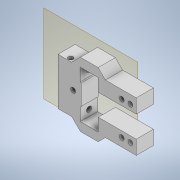
# Autodesk Inventor part: 30_Cube_Cube_Z_Focus_MGN_NEMA_belt_pushing_slide_v3
Saved by Autodesk Inventor 2022 (Build 260153000, 153)
## iProperties
Created: 2021-12-20
Part Number: 30_Cube_Cube_Z_Focus_MGN_NEMA_belt_pushing_slide_v3
Material: Generisch
Document SubType Name: Modeling
Designer: diederichbenedict
Density: 1 g/cm^3
Appearance: Vorgabe
Author: diederichbenedict
Autodesk Inventor part; units mm, degrees
ref_plane "YZ Plane" through (0, 0, 0) normal (1, 0, 0) x (0, 1, 0)
ref_plane "XZ Plane" through (0, 0, 0) normal (0, 1, 0) x (-1, 0, 0)
ref_plane "XY Plane" through (0, 0, 0) normal (0, 0, 1) x (1, 0, 0)
ref_plane "Arbeitsebene1" through (0, 0, 0) normal (0, 0, 1) x (1, 0, 0)
sketch "Skizze1" plane through (0, 0, 0) normal (0, 0, 1) x (1, 0, 0)
  arc A0 (12.7966, 13.5152) -> (12.2972, 14.0928) centre (11.6862, 13.06) ccw construction
  arc A1 (12.1755, 14.2862) -> (12.2972, 14.0928) centre (12.4245, 14.308) ccw construction
  line L0 (12.1755, 14.2862) -> (12.1453, 14.6318) construction
  arc A2 (12.1453, 14.6318) -> (11.8962, 14.86) centre (11.8962, 14.61) ccw construction
  line L1 (11.8962, 14.86) -> (11.4438, 14.86) construction
  arc A3 (11.4438, 14.86) -> (11.1947, 14.6318) centre (11.4438, 14.61) ccw construction
  line L2 (11.1947, 14.6318) -> (11.1627, 14.2652) construction
  arc A4 (11.0468, 14.0755) -> (11.1627, 14.2652) centre (10.9136, 14.287) ccw construction
  arc A5 (11.0468, 14.0755) -> (10.5759, 13.5152) centre (11.6862, 13.06) ccw construction
  arc A6 (10.3446, 13.36) -> (10.5759, 13.5152) centre (10.3446, 13.61) ccw construction
  line L3 (10.3446, 13.36) -> (9.67, 13.36) construction
  line L4 (9.67, 13.36) -> (9.17, 13.86) construction
  line L5 (9.17, 13.86) -> (9.17, 24.86) construction
  line L6 (9.17, 24.86) -> (9.67, 25.36) construction
  line L7 (9.67, 25.36) -> (10.3446, 25.36) construction
  arc A7 (10.5759, 25.2048) -> (10.3446, 25.36) centre (10.3446, 25.11) ccw construction
  arc A8 (10.5759, 25.2048) -> (11.0468, 24.6445) centre (11.6862, 25.66) ccw construction
  arc A9 (11.1627, 24.4548) -> (11.0468, 24.6445) centre (10.9136, 24.433) ccw construction
  line L8 (11.1627, 24.4548) -> (11.1947, 24.0882) construction
  arc A10 (11.1947, 24.0882) -> (11.4438, 23.86) centre (11.4438, 24.11) ccw construction
  line L9 (11.4438, 23.86) -> (11.8962, 23.86) construction
  arc A11 (11.8962, 23.86) -> (12.1453, 24.0882) centre (11.8962, 24.11) ccw construction
  line L10 (12.1453, 24.0882) -> (12.1755, 24.4338) construction
  arc A12 (12.2972, 24.6272) -> (12.1755, 24.4338) centre (12.4245, 24.412) ccw construction
  arc A13 (12.2972, 24.6272) -> (12.7966, 25.2048) centre (11.6862, 25.66) ccw construction
  arc A14 (13.0279, 25.36) -> (12.7966, 25.2048) centre (13.0279, 25.11) ccw construction
  line L11 (13.0279, 25.36) -> (14.17, 25.36) construction
  line L12 (14.17, 25.36) -> (14.17, 32.26) construction
  line L13 (14.17, 32.26) -> (13.57, 32.86) construction
  line L14 (13.57, 32.86) -> (10.17, 32.86) construction
  arc A15 (9.37, 32.86) -> (10.17, 32.86) centre (9.77, 33.16) ccw construction
  line L15 (9.37, 32.86) -> (4.77, 32.86) construction
  line L16 (4.77, 32.86) -> (4.17, 32.26) construction
  line L17 (4.17, 32.26) -> (4.17, 25.76) construction
  line L18 (4.17, 25.76) -> (4.57, 25.36) construction
  line L19 (4.57, 25.36) -> (4.57, 13.36) construction
  line L20 (4.57, 13.36) -> (4.17, 12.96) construction
  line L21 (4.17, 12.96) -> (4.17, 6.46) construction
  line L22 (4.17, 6.46) -> (4.77, 5.86) construction
  line L23 (4.77, 5.86) -> (13.57, 5.86) construction
  line L24 (13.57, 5.86) -> (14.17, 6.46) construction
  line L25 (14.17, 6.46) -> (14.17, 13.36) construction
  line L26 (14.17, 13.36) -> (13.0279, 13.36) construction
  arc A16 (12.7966, 13.5152) -> (13.0279, 13.36) centre (13.0279, 13.61) ccw construction
  line L27 (13.6528, 5.66) -> (4.6872, 5.66) construction
  line L28 (4.6872, 5.66) -> (3.97, 6.3772) construction
  line L29 (3.97, 6.3772) -> (3.97, 13.0428) construction
  line L30 (3.97, 13.0428) -> (4.37, 13.4428) construction
  line L31 (4.37, 13.4428) -> (4.37, 25.2772) construction
  line L32 (4.37, 25.2772) -> (3.97, 25.6772) construction
  line L33 (3.97, 25.6772) -> (3.97, 32.3428) construction
  line L34 (3.97, 32.3428) -> (4.6872, 33.06) construction
  line L35 (4.6872, 33.06) -> (9.4872, 33.06) construction
  arc A17 (9.4872, 33.06) -> (10.0528, 33.06) centre (9.77, 33.16) ccw construction
  line L36 (10.0528, 33.06) -> (13.6528, 33.06) construction
  line L37 (13.6528, 33.06) -> (14.37, 32.3428) construction
  line L38 (14.37, 32.3428) -> (14.37, 25.16) construction
  line L39 (14.37, 25.16) -> (13.0279, 25.16) construction
  arc A18 (13.0279, 25.16) -> (12.9816, 25.129) centre (13.0279, 25.11) ccw construction
  arc A19 (12.3991, 24.4551) -> (12.9816, 25.129) centre (11.6862, 25.66) ccw construction
  arc A20 (12.3991, 24.4551) -> (12.3747, 24.4164) centre (12.4245, 24.412) ccw construction
  line L40 (12.3747, 24.4164) -> (12.3445, 24.0708) construction
  arc A21 (11.8962, 23.66) -> (12.3445, 24.0708) centre (11.8962, 24.11) ccw construction
  line L41 (11.8962, 23.66) -> (11.4438, 23.66) construction
  arc A22 (10.9955, 24.0708) -> (11.4438, 23.66) centre (11.4438, 24.11) ccw construction
  line L42 (10.9955, 24.0708) -> (10.9634, 24.4373) construction
  arc A23 (10.9634, 24.4373) -> (10.9403, 24.4753) centre (10.9136, 24.433) ccw construction
  arc A24 (10.3909, 25.129) -> (10.9403, 24.4753) centre (11.6862, 25.66) ccw construction
  arc A25 (10.3909, 25.129) -> (10.3446, 25.16) centre (10.3446, 25.11) ccw construction
  line L43 (10.3446, 25.16) -> (9.7528, 25.16) construction
  line L44 (9.7528, 25.16) -> (9.37, 24.7772) construction
  line L45 (9.37, 24.7772) -> (9.37, 13.9428) construction
  line L46 (9.37, 13.9428) -> (9.7528, 13.56) construction
  line L47 (9.7528, 13.56) -> (10.3446, 13.56) construction
  arc A26 (10.3446, 13.56) -> (10.3909, 13.591) centre (10.3446, 13.61) ccw construction
  arc A27 (10.9403, 14.2447) -> (10.3909, 13.591) centre (11.6862, 13.06) ccw construction
  arc A28 (10.9403, 14.2447) -> (10.9634, 14.2827) centre (10.9136, 14.287) ccw construction
  line L48 (10.9634, 14.2827) -> (10.9955, 14.6492) construction
  arc A29 (11.4438, 15.06) -> (10.9955, 14.6492) centre (11.4438, 14.61) ccw construction
  line L49 (11.4438, 15.06) -> (11.8962, 15.06) construction
  arc A30 (12.3445, 14.6492) -> (11.8962, 15.06) centre (11.8962, 14.61) ccw construction
  line L50 (12.3445, 14.6492) -> (12.3747, 14.3036) construction
  arc A31 (12.3747, 14.3036) -> (12.3991, 14.2649) centre (12.4245, 14.308) ccw construction
  arc A32 (12.9816, 13.591) -> (12.3991, 14.2649) centre (11.6862, 13.06) ccw construction
  arc A33 (12.9816, 13.591) -> (13.0279, 13.56) centre (13.0279, 13.61) ccw construction
  line L51 (13.0279, 13.56) -> (14.37, 13.56) construction
  line L52 (14.37, 13.56) -> (14.37, 6.3772) construction
  line L53 (14.37, 6.3772) -> (13.6528, 5.66) construction
  line L54 (16.97, 24.8315) -> (24.85, 24.8315) construction
  line L55 (24.85, 36.23) -> (20.77, 36.23) construction
  line L56 (20.77, 36.23) -> (16.87, 36.23) construction
  line L57 (14.37, 25.66) -> (36.4731, 25.66)
  line L58 (14.37, 25.66) -> (36.4731, 25.66) construction
  line L59 (36.4731, 25.66) -> (36.4731, 33.86)
  line L60 (36.4731, 33.86) -> (18.5197, 33.86)
  line L61 (18.5197, 33.86) -> (14.3197, 38.06)
  line L62 (14.3197, 38.06) -> (3.97, 38.06)
  line L63 (-9.03, 33.06) -> (-9.03, 19.36)
  line L64 (-9.03, 19.36) -> (4.37, 19.36)
  line L65 (4.37, 19.36) -> (4.37, 25.2772)
  line L66 (4.37, 25.2772) -> (3.97, 25.6772)
  line L67 (3.97, 25.6772) -> (3.97, 33.06)
  line L68 (3.97, 33.06) -> (14.37, 33.06)
  line L69 (14.37, 33.06) -> (14.37, 25.66)
  circle A34 centre (-3.43, 19.36) radius 1.75 construction
  circle A35 centre (-0.2031, 19.36) radius 1.4
  circle A36 centre (60.62, 30.4425) radius 2.45 projected
  circle A37 centre (35.7803, 19.36) radius 2.45 projected
  circle A38 centre (60.62, 8.3286) radius 2.45 projected
  line L70 (29.0574, 13.415) -> (26.7455, 13.415) projected
  line L71 (26.7455, 13.415) -> (26.7455, 10.1303) projected
  arc A39 (26.7455, 9.327) -> (26.7455, 10.1303) centre (28.0867, 9.7286) ccw projected
  line L72 (26.7455, 9.327) -> (26.7455, 5.8628) projected
  line L73 (26.7455, 5.8628) -> (35.12, 4.36) projected
  line L74 (35.12, 4.36) -> (65.12, 4.36) projected
  line L75 (65.12, 4.36) -> (65.12, 34.36) projected
  line L76 (65.12, 34.36) -> (35.12, 34.36) projected
  line L77 (35.12, 34.36) -> (26.7455, 32.9029) projected
  line L78 (26.7455, 32.9029) -> (26.7455, 29.4442) projected
  arc A40 (26.7455, 28.6409) -> (26.7455, 29.4442) centre (28.0867, 29.0425) ccw projected
  line L79 (26.7455, 28.6409) -> (26.7455, 25.3561) projected
  line L80 (26.7455, 25.3561) -> (29.0574, 25.3561) projected
  line L81 (29.0574, 25.3561) -> (29.0574, 13.415) projected
  circle A41 centre (50.12, 19.36) radius 10.5 projected
  circle A42 centre (33.0867, 29.0425) radius 1.4 projected
  circle A43 centre (33.0867, 9.7286) radius 1.4 projected
  line L82 (36.7731, 34.36) -> (36.7731, 25.3561) projected
  line L83 (36.7731, 13.415) -> (36.7731, 4.36) projected
  circle A44 centre (33.0867, 29.0425) radius 1.4
  circle A45 centre (28.0867, 29.0425) radius 1.4
  line L84 (3.97, 38.06) -> (-1.03, 33.06)
  line L85 (3.97, 38.06) -> (11.0411, 38.06) construction
  line L86 (-1.03, 33.06) -> (-9.03, 33.06)
  point P0 (0, 0)
  point P1 (1.1969, 19.36)
  point P2 (-1.6031, 19.36)
  dimension "d0" = 0.2
  dimension "d2" = 5
  dimension "d4" = 13
  dimension "d5" = 2.8
  dimension "d7" = 0.5
  dimension "d8" = 3.5
  dimension "d19" = 0.3
  dimension "d20" = 0.5
  dimension "d21" = 135
  dimension "d28" = 8.8269
  constraints: 86 end point, 36 point on circle, 20 centre point, 6 parallel, 5 point on line, 2 coincident, 2 concentric, 2 equal length, 2 horizontal, 2 perpendicular, 1 collinear, 1 midpoint, 1 vertical, 43 other
  measures "d0" distance between parallel lines of L23 L27
  measures "d2" distance between parallel lines of L35 L62
  measures "d4" distance between parallel lines of L67 L63
  measures "d5" diameter of A35
  measures "d7" distance from line of L57 L38.end
  measures "d8" distance from line of L68.end L61
  measures "d19" distance between parallel lines of L82 L59
  measures "d20" distance between parallel lines of L76 L60
  measures "d21" angle of L84 L85
  measures "d28" distance of A35.centre L63.end
extrude "Extrusion1" add sketch "Skizze1" along normal blind 10 contours L69 L68 L67 L66 L65 L64 A35 L63 L86 L84 L62 L61 L60 L77 L78 A45 L79 L57 | L79 A40 L78 L77 L60 L59 L57
sketch "Skizze2" plane through (-9.03, 19.36, 0) normal (-1, 0, 0) x (0, 0, 1)
  circle A0 centre (12.1869, 10) radius 1.75 projected
  line L0 (0, 13.7) -> (0, 0) projected
  line L1 (0, 0) -> (10, 0) projected
  line L2 (10, 13.7) -> (10, 0) projected
  line L3 (0, 13.7) -> (10, 13.7) projected
  circle A1 centre (5, 10) radius 1.5
  point P0 (0, -19.36)
  dimension "d11" = 3
  constraints: 1 centre point
  measures "d11" diameter of A1
hole "Bohrung1" at (-9.03, 29.36, 5) direction (1, 0, 0) diameter 3 depth 20 tip angle 118 counterbore diameter 6 counterbore depth 4
sketch "Skizze3" plane through (-9.03, 33.06, 0) normal (0, 1, 0) x (1, 0, 0)
  line L0 (4.1, -9.9) -> (4.1, 19.6933)
  line L1 (7.1, -9.9) -> (7.1, 19.6933)
  circle A0 centre (5.5663, -8.2216) radius 1.4
  point P0 (9.03, 0)
  dimension "d22" = 2.8
  constraints: 4 end point, 2 vertical, 1 centre point, 4 other
  measures "d22" diameter of A0
extrude "Extrusion2" cut sketch "Skizze3" against normal blind 10
mirror "Spiegeln2" about plane through (-9.03, 19.36, 0) normal (0, -1, 0) of "Extrusion1", "Bohrung1", "Extrusion2"
sketch "Skizze4" plane through (0, 0, 0) normal (0, 0, -1) x (-1, 0, 0)
  circle A0 centre (0.2031, 19.36) radius 1.4 projected
  circle A1 centre (-28.0867, 9.6775) radius 1.4 projected
  circle A2 centre (-33.0867, 9.6775) radius 1.4 projected
  line L0 (-4.37, 13.4428) -> (-4.37, 25.2772) projected
  line L1 (-4.37, 13.4428) -> (-3.97, 13.0428) projected
  line L2 (-3.97, 13.0428) -> (-3.97, 5.66) projected
  line L3 (-3.97, 5.66) -> (-14.37, 5.66) projected
  line L4 (-14.37, 5.66) -> (-14.37, 13.06) projected
  line L5 (-14.37, 13.06) -> (-36.4731, 13.06) projected
  line L6 (-36.4731, 13.06) -> (-36.4731, 4.86) projected
  line L7 (-36.4731, 4.86) -> (-18.5197, 4.86) projected
  line L8 (-18.5197, 4.86) -> (-14.3197, 0.66) projected
  line L9 (-14.3197, 0.66) -> (-3.97, 0.66) projected
  line L10 (-3.97, 0.66) -> (1.03, 5.66) projected
  line L11 (1.03, 5.66) -> (9.03, 5.66) projected
  line L12 (9.03, 33.06) -> (9.03, 5.66) projected
  line L13 (1.03, 33.06) -> (9.03, 33.06) projected
  line L14 (-3.97, 38.06) -> (1.03, 33.06) projected
  line L15 (-14.3197, 38.06) -> (-3.97, 38.06) projected
  line L16 (-18.5197, 33.86) -> (-14.3197, 38.06) projected
  line L17 (-36.4731, 33.86) -> (-18.5197, 33.86) projected
  line L18 (-36.4731, 25.66) -> (-36.4731, 33.86) projected
  line L19 (-14.37, 25.66) -> (-36.4731, 25.66) projected
  line L20 (-14.37, 33.06) -> (-14.37, 25.66) projected
  line L21 (-3.97, 33.06) -> (-14.37, 33.06) projected
  line L22 (-3.97, 25.6772) -> (-3.97, 33.06) projected
  line L23 (-4.37, 25.2772) -> (-3.97, 25.6772) projected
  circle A3 centre (-33.0867, 29.0425) radius 1.4 projected
  circle A4 centre (-28.0867, 29.0425) radius 1.4 projected
  line L24 (-3.2969, 21.3807) -> (0.2031, 23.4015)
  line L25 (0.2031, 23.4015) -> (3.7031, 21.3807)
  line L26 (3.7031, 21.3807) -> (3.7031, 17.3393)
  line L27 (3.7031, 17.3393) -> (0.2031, 15.3185)
  line L28 (0.2031, 15.3185) -> (-3.2969, 17.3393)
  line L29 (-3.2969, 17.3393) -> (-3.2969, 21.3807)
  point P0 (0, 0)
  dimension "d25" = 7
  constraints: 12 end point, 1 coincident, 1 parallel, 13 other
  measures "d25" distance between parallel lines of L24 L27
extrude "Extrusion3" cut sketch "Skizze4" against normal blind 5 contours A0 | L24 L25 L26 L27 L28 L29
